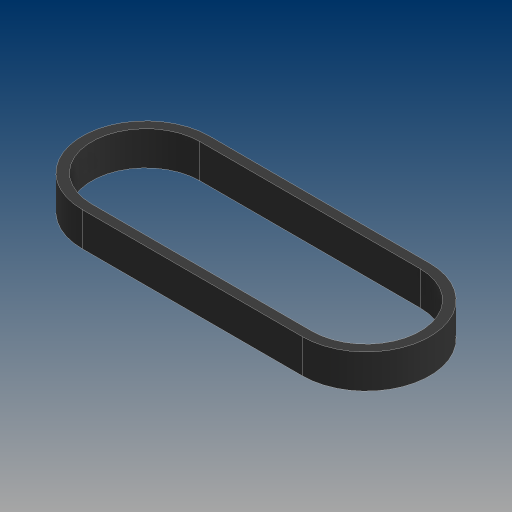
# Autodesk Inventor part: INTK_013_Belt5
Saved by Autodesk Inventor 2024.3 (Build 283343000, 343)
## iProperties
Created: 2024-08-07
Part Number: INTK_013_Belt5
Material: Rubber, Silicone
Document SubType Name: Modeling
Designer: Kenji
Density: 1.25 g/cm^3
Appearance: Rubber - Black
Author: Kenji
Autodesk Inventor part; units mm, degrees
ref_plane "YZ Plane" through (0, 0, 0) normal (1, 0, 0) x (0, 1, 0)
ref_plane "XZ Plane" through (0, 0, 0) normal (0, 1, 0) x (-1, 0, 0)
ref_plane "XY Plane" through (0, 0, 0) normal (0, 0, 1) x (1, 0, 0)
sketch "Sketch1" plane through (0, 0, 0) normal (0, 1, 0) x (-1, 0, 0)
  circle A0 centre (0, 0) radius 14.3256 construction
  line L0 (0, 0) -> (58.3628, 0) construction
  circle A1 centre (58.3628, 0) radius 14.3256 construction
  line L1 (58.3628, 14.3256) -> (0, 14.3256)
  line L2 (58.3628, -14.3256) -> (0, -14.3256)
  arc A2 (58.3628, -14.3256) -> (58.3628, 14.3256) centre (58.3628, 0) ccw
  arc A3 (0, 14.3256) -> (0, -14.3256) centre (0, 0) ccw
  line L3 (0, 16.8656) -> (58.3628, 16.8656)
  arc A4 (58.3628, -16.8656) -> (58.3628, 16.8656) centre (58.3628, 0) ccw
  line L4 (58.3628, -16.8656) -> (0, -16.8656)
  arc A5 (0, 16.8656) -> (0, -16.8656) centre (0, 0) ccw
  dimension "d0" = 28.6512
  dimension "d1" = 58.3628
  dimension "d2" = 28.6512
  dimension "d3" = 2.54
  constraints: 12 point on circle, 10 end point, 7 tangent, 6 centre point, 2 coincident, 1 horizontal, 3 other
  measures "d0" diameter of A0
  measures "d1" distance of L0.start L0.end
  measures "d2" diameter of A1
  measures "d3" distance between parallel lines of L3 L1
extrude "Extrusion1" add sketch "Sketch1" along normal blind 8.9916
body "Solid1"
